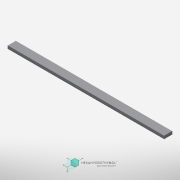
# Autodesk Inventor part: MPX-side-spacer
Saved by Autodesk Inventor 2016 (Build 200138000, 138)
## iProperties
Created: 2015-05-28
Part Number: MPX-side-spacer
Material: Wood (Walnut)
Document SubType Name: Modeling
Designer: as
Mass: 257.4 g
Surface Area: 870 cm^2
Volume: 468 cm^3
Density: 0.55 g/cm^3
Appearance: Walnut - Natural Polished
Author: as
Autodesk Inventor part; units mm, degrees
ref_plane "YZ Plane" through (0, 0, 0) normal (1, 0, 0) x (0, 1, 0)
ref_plane "XZ Plane" through (0, 0, 0) normal (0, 1, 0) x (-1, 0, 0)
ref_plane "XY Plane" through (0, 0, 0) normal (0, 0, 1) x (1, 0, 0)
sketch "Sketch1" plane through (0, 0, 0) normal (0, 0, 1) x (1, 0, 0)
  line L0 (0, 0) -> (780, 0)
  line L1 (780, 0) -> (780, 40)
  line L2 (780, 40) -> (0, 40)
  line L3 (0, 40) -> (0, 0)
  dimension "d0" = 40
  constraints: 8 end point, 2 parallel, 1 horizontal, 1 perpendicular
  measures "d0" distance of L1.end L0.end
extrude "Extrusion1" add sketch "Sketch1" along normal blind 15
body "Solid1"
